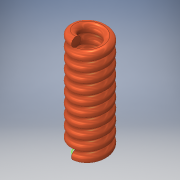
# Autodesk Inventor part: Sun_Coil
Saved by Autodesk Inventor 2016 (Build 200138000, 138)
## iProperties
Created: 2017-11-25
Part Number: Sun_Coil
Material: Generic
Document SubType Name: Modeling
Designer: Titus
Density: 1 g/cm^3
Appearance: Copper - Satin
Mass: 0.51627 g
Surface Area: 8.79555 cm^2
Volume: 0.51627 cm^3
Author: Titus
Autodesk Inventor part; units mm, degrees
ref_plane "YZ Plane" through (0, 0, 0) normal (1, 0, 0) x (0, 1, 0)
ref_plane "XZ Plane" through (0, 0, 0) normal (0, 1, 0) x (-1, 0, 0)
ref_plane "XY Plane" through (0, 0, 0) normal (0, 0, 1) x (1, 0, 0)
sketch "Sketch3" plane through (0, 0, 0) normal (0, 0, 1) x (1, 0, 0)
  circle A0 centre (0, 0) radius 1.1662
  constraints: 1 centre point, 1 coincident
sketch "Sketch4" plane through (0, 0, 0) normal (1, 0, 0) x (0, 1, 0)
  line L0 (0, 0) -> (0, -3.6254) construction
  line L1 (0, -3.6254) -> (26.9181, -3.6254)
  circle A0 centre (0, 0) radius 1.2012
  dimension "d10" = 26.9181
  constraints: 4 end point, 1 centre point, 1 coincident, 1 horizontal, 1 perpendicular, 1 vertical, 1 other
  measures "d10" distance of L0.end L1.end
coil "Coil1" sketch "Sketch4" operation add axis through (0, 0, -3.6254) along (0, 1, 0) pitch 2.54 turns 10 hand right
body "Solid2"
